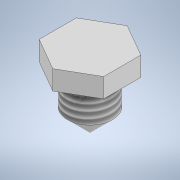
# Autodesk Inventor part: side bolt
Saved by Autodesk Inventor 2021 (Build 250183000, 183)
## iProperties
Created: 2021-02-27
Part Number: side bolt
Material: Generic
Document SubType Name: Modeling
Designer: WASHINGTON
Density: 1 g/cm^3
Appearance: Default
Author: WASHINGTON
Autodesk Inventor part; units mm, degrees
ref_plane "YZ Plane" through (0, 0, 0) normal (1, 0, 0) x (0, 1, 0)
ref_plane "XZ Plane" through (0, 0, 0) normal (0, 1, 0) x (-1, 0, 0)
ref_plane "XY Plane" through (0, 0, 0) normal (0, 0, 1) x (1, 0, 0)
sketch "Sketch1" plane through (0, 0, 0) normal (1, 0, 0) x (0, 1, 0)
  line L0 (0, 0) -> (8.5, 0)
  line L1 (8.5, 0) -> (8.5, 3.5)
  line L2 (8.5, 3.5) -> (3.5, 3.5)
  line L3 (3.5, 3.5) -> (0, 0)
  dimension "d0" = 135
  dimension "d1" = 3.5
  dimension "d2" = 8.5
  constraints: 8 end point, 2 perpendicular, 1 horizontal
  measures "d0" angle of L3 L2
  measures "d1" distance of L0.end L1.end
  measures "d2" distance from line of L0.start L1
revolve "Revolution1" add sketch "Sketch1" angle 360 about axis through (0, 0, 0) along (0, 1, 0)
thread "Thread1" size "M7x1" class "6g" standard "ANSI Metric M Profile" full length
sketch "Sketch2" plane through (0, 8.5, 0) normal (0, 1, 0) x (1, 0, 0)
  circle A0 centre (0, 0) radius 5 construction
  line L0 (-5, -2.8868) -> (-5, 2.8868)
  line L1 (-5, 2.8868) -> (0, 5.7735)
  line L2 (0, 5.7735) -> (5, 2.8868)
  line L3 (5, 2.8868) -> (5, -2.8868)
  line L4 (5, -2.8868) -> (0, -5.7735)
  line L5 (0, -5.7735) -> (-5, -2.8868)
  dimension "d6" = 10
  dimension "d7" = 120
  constraints: 12 end point, 5 tangent, 3 equal length, 1 centre point, 1 coincident, 1 parallel, 1 vertical, 1 vertical alignment
  measures "d6" diameter of A0
  measures "d7" angle of L3 L4
extrude "Extrusion1" add sketch "Sketch2" along normal blind 3
body "Solid1"
